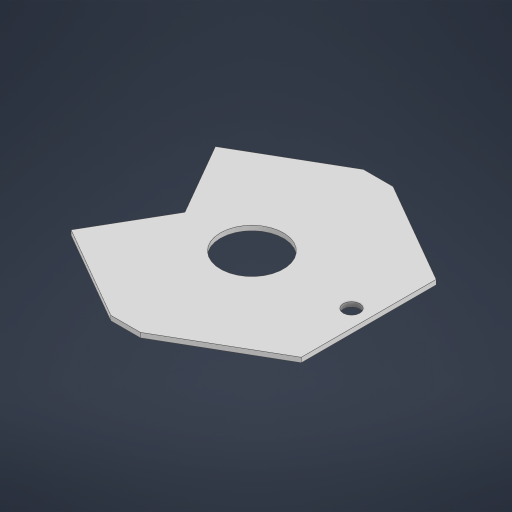
# Autodesk Inventor part: PCB
Saved by Autodesk Inventor 2023 (Build 270158000, 158)
## iProperties
Created: 2022-10-19
Part Number: PCB
Material: Generic
Document SubType Name: Modeling
Designer: jevan
Density: 1 g/cm^3
Appearance: Default
Author: jevan
Autodesk Inventor part; units mm, degrees
ref_plane "YZ Plane" through (0, 0, 0) normal (1, 0, 0) x (0, 1, 0)
ref_plane "XZ Plane" through (0, 0, 0) normal (0, 1, 0) x (-1, 0, 0)
ref_plane "XY Plane" through (0, 0, 0) normal (0, 0, 1) x (1, 0, 0)
sketch "Sketch1" plane through (0, 0, 0) normal (0, 1, 0) x (-1, 0, 0)
  circle A0 centre (0, 0) radius 6.625
  line L0 (0, -28.4345) -> (-24.625, -14.2173)
  line L1 (-24.625, -14.2173) -> (-24.625, 14.2173)
  line L2 (-24.625, 14.2173) -> (0, 28.4345)
  line L3 (0, 28.4345) -> (24.625, 14.2173)
  line L4 (24.625, 14.2173) -> (24.625, -14.2173)
  line L5 (24.625, -14.2173) -> (0, -28.4345)
  line L6 (22.9063, 15.2096) -> (14.125, 0)
  line L7 (14.125, 0) -> (22.9062, -15.2096)
  line L8 (14.125, 0) -> (24.625, 0)
  line L9 (3.1177, 26.6345) -> (-3.1177, 26.6345)
  line L10 (3.1177, -26.6345) -> (-3.1177, -26.6345)
  circle A1 centre (-21, 0) radius 1.75
  line L11 (0, 0) -> (-21, 0)
  dimension "d0" = 13.25
  dimension "d1" = 49.25
  dimension "d4" = 120
  dimension "d5" = 120
  dimension "d6" = 10.5
  dimension "d7" = 24.625
  dimension "d8" = 1.8
  dimension "d9" = 1.8
  dimension "d10" = 3.5
  dimension "d11" = 21
  constraints: 24 end point, 7 point on line, 3 equal length, 3 parallel, 3 perpendicular, 2 centre point, 2 horizontal, 1 coincident, 1 midpoint, 1 vertical
  measures "d0" diameter of A0
  measures "d1" distance between parallel lines of L1 L4
  measures "d4" angle of L2 L3
  measures "d5" angle of L1 L2
  measures "d6" distance from line of L6.end L4
  measures "d7" distance from line of point (0, 0) L4
  measures "d8" distance from line of L2.end L9
  measures "d9" distance from line of L0.start L10
  measures "d10" diameter of A1
  measures "d11" distance of L11.end point (0, 0)
extrude "Extrusion1" add sketch "Sketch1" along normal blind 1 contours L0 L1 L2 L9 L3 L6 L7 L5 L10 | A1
extrude "Extrusion2" cut sketch "Sketch1" along normal through all contours A1
body "Solid1"
